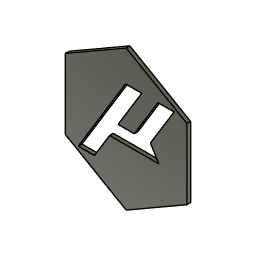
ParametricLogo (Autodesk Fusion 360 design; units mm, degrees)
Autodesk Fusion 360 part; units mm, degrees
sketch "Sketch3" plane through (0, 0, 0) normal (0, 1, 0) x (1, 0, 0)
  line L0 (50, 28.8675) -> (0, 57.735)
  line L1 (0, 57.735) -> (-50, 28.8675)
  line L2 (-50, 28.8675) -> (-50, -28.8675)
  line L3 (-50, -28.8675) -> (0, -57.735)
  line L4 (0, -57.735) -> (50, -28.8675)
  line L5 (50, -28.8675) -> (50, 28.8675)
  line L6 (47.3, 27.3087) -> (0, 54.6173) construction
  line L7 (0, 54.6173) -> (-47.3, 27.3087) construction
  line L8 (-47.3, 27.3087) -> (-47.3, -27.3087) construction
  line L9 (-47.3, -27.3087) -> (0, -54.6173) construction
  line L10 (0, -54.6173) -> (47.3, -27.3087) construction
  line L11 (47.3, -27.3087) -> (47.3, 27.3087) construction
  line L12 (50, -28.8675) -> (-50, -28.8675) construction
  line L13 (0, 0) -> (50, 0) construction
  line L14 (0, -57.735) -> (0, -31.867) construction
  line L15 (0, -31.867) -> (-0.479, -31.867) construction
  line L16 (50, -31.8675) -> (-50, -31.8675) construction
  line L17 (50, 31.8675) -> (-50, 31.8675) construction
  line L18 (-0.479, -31.867) -> (-39.4038, 31.8675)
  line L19 (-0.479, -31.867) -> (12.815, -31.867)
  line L20 (0, 0) -> (-47.3, 0) construction
  line L21 (12.815, -31.867) -> (-6.6473, 0)
  line L22 (-6.6473, 0) -> (6.6467, 0)
  line L23 (6.6467, 0) -> (26.1093, -31.8675)
  line L24 (26.1093, -31.8675) -> (39.4033, -31.8675)
  line L25 (39.4033, -31.8675) -> (19.9407, 0)
  line L26 (-6.6473, 0) -> (-13.5763, 11.3454) construction
  line L27 (-39.4038, 31.8675) -> (-26.1098, 31.8675)
  line L28 (-26.1098, 31.8675) -> (-13.5763, 11.3454)
  line L29 (19.9407, 0) -> (39.4033, -31.8675) construction
  line L30 (39.4033, 31.8675) -> (19.9407, 0) construction
  line L31 (-13.5763, 11.3454) -> (26.8698, 11.3454)
  line L32 (26.8698, 11.3454) -> (19.9407, 0)
  dimension "d2" = 50
  dimension "d9" = 25.868
  dimension "d12" = 0.479
  dimension "d14" = 13.294
  constraint coincident L13.start L20.start
  constraint vertical L5
  constraint midpoint L5 L13.end
  constraint vertical L14
  constraint perpendicular L14 L15
  constraint symmetric L13 L16.start L17.start
  constraint symmetric L13 L16.end L17.end
  constraint coincident L7 L18.end
  constraint coincident L17 L18.end
  constraint parallel L16 L19
  constraint midpoint L8 L20.end
  constraint coincident L20 L21.end
  constraint parallel L18 L21
  constraint coincident L13 L22.end
  constraint parallel L13 L22
  constraint equal L19 L22
  constraint coincident L16 L23.end
  constraint parallel L21 L23
  constraint coincident L16 L24.end
  constraint equal L19 L24
  constraint coincident L13 L25.end
  constraint parallel L23 L25
  constraint parallel L21 L26
  constraint equal L24 L26
  constraint coincident L17 L27.end
  constraint equal L24 L27
  constraint symmetric L13 L24.end L30.start
  constraint symmetric L13 L25.end L29.start
  constraint coincident L30 L31.end
  constraint horizontal L31
  measures "d2" distance of L13.start L5
  measures "d9" distance of L3.end L14.end
  measures "d12" distance of L14.end L15.end
  measures "d14" distance of L15.end L19.end
extrude "Extrude1" add sketch "Sketch3" along normal blind 3
equation "logoA = 100 mm"
equation "d2 = logoA / 2"
equation "logoB = 0.125 * logoA"
equation "logoC = 0.03 * logoA"
equation "logoD = 0.027 * logoA"
equation "d6 = -logoD"
equation "logoE = 0.25868 * logoA"
equation "d9 = logoE"
equation "d12 = 0.00479 * logoA"
equation "d13 = -logoC"
equation "d14 = 0.13294 * logoA"
